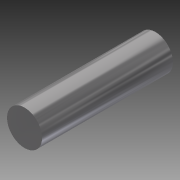
# Autodesk Inventor part: shortEndAxel
Saved by Autodesk Inventor 2013 (Build 170138000, 138)
## iProperties
Created: 2013-02-24
Part Number: shortEndAxel
Material: Steel, Alloy
Document SubType Name: Modeling
Designer: Nano
Density: 7.85 g/cm^3
Mass: 44.2017 g
Surface Area: 20.2683 cm^2
Volume: 5.63079 cm^3
d0: 0.469 in
d1: 1.750 in
d2: 0.00 deg
Author: Nano
Autodesk Inventor part; units mm, degrees
ref_plane "YZ Plane" through (0, 0, 0) normal (1, 0, 0) x (0, 1, 0)
ref_plane "XZ Plane" through (0, 0, 0) normal (0, 1, 0) x (-1, 0, 0)
ref_plane "XY Plane" through (0, 0, 0) normal (0, 0, 1) x (1, 0, 0)
sketch "Sketch1" plane through (0, 0, 0) normal (0, 0, 1) x (1, 0, 0)
  circle A0 centre (0, 0) radius 5.9531
  dimension "d0" = 11.9062
  dimension "d0" = 11.9062
  constraints: 1 centre point
  measures "d0" diameter of A0
extrude "Extrusion1" add sketch "Sketch1" along normal blind 44.45
body "Solid1"
